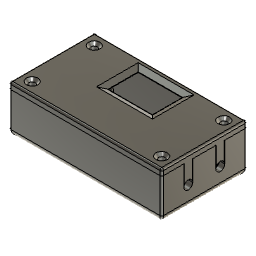
Controller_DC-DC_box (Autodesk Fusion 360 design; units mm, degrees)
Autodesk Fusion 360 part; units mm, degrees
sketch "Sketch1" plane through (0, 0, 0) normal (0, 0, 1) x (1, 0, 0)
  line L0 (-40, 21) -> (40, 21)
  line L1 (40, 21) -> (40, -21)
  line L2 (40, -21) -> (-40, -21)
  line L3 (-40, -21) -> (-40, 21)
  line L4 (1.75, 0) -> (22.5, 0)
  line L5 (0, 1.75) -> (0, 22.5)
  dimension "d1" = 80
  dimension "d2" = 42
  constraint horizontal L0
  constraint vertical L1
  constraint horizontal L2
  constraint vertical L3
  constraint symmetric L0 L2 L4
  constraint symmetric L1 L3 L5
  measures "d1" distance of L0.start L0.end
  measures "d2" distance of L0.start L2.end
extrude "Extrude1" add sketch "Sketch1" along normal blind 3 makes body 1
sketch "Sketch2" plane through (0, 0, 0) normal (0, 0, -1) x (1, 0, 0)
  line L0 (40, 21) -> (-40, 21)
  line L1 (-40, 21) -> (-40, -21)
  line L2 (-40, -21) -> (40, -21)
  line L3 (40, -21) -> (40, 21)
  line L4 (-43, -24) -> (43, -24)
  line L5 (43, -24) -> (43, 24)
  line L6 (43, 24) -> (-43, 24)
  line L7 (-43, 24) -> (-43, -24)
  dimension "d5" = 3
extrude "Extrude2" add sketch "Sketch2" against normal blind 23 bodies 1
sketch "Sketch3" plane through (0, 0, 3) normal (0, 0, 1) x (-1, 0, 0)
  line L0 (40, 21) -> (-40, 21)
  line L1 (-40, 21) -> (-40, -21)
  line L2 (-40, -21) -> (40, -21)
  line L3 (40, -21) -> (40, 21)
  line L4 (29, -16) -> (-29, -16) construction
  line L5 (-29, -16) -> (-29, 16) construction
  line L6 (-29, 16) -> (29, 16) construction
  line L7 (29, 16) -> (29, -16) construction
  line L8 (-1.75, 0) -> (-22.5, 0) construction
  line L9 (0, -1.75) -> (0, -22.5) construction
  circle A0 centre (29, -16) radius 3.5
  circle A1 centre (29, -16) radius 1.75
  circle A2 centre (-29, -16) radius 1.75
  circle A3 centre (-29, -16) radius 3.5
  circle A4 centre (-29, 16) radius 1.75
  circle A5 centre (-29, 16) radius 3.5
  circle A6 centre (29, 16) radius 1.75
  circle A7 centre (29, 16) radius 3.5
  dimension "d8" = 58
  dimension "d9" = 32
  dimension "d10" = 7
  dimension "d11" = 3.5
  constraint horizontal L4
  constraint vertical L5
  constraint horizontal L6
  constraint vertical L7
  constraint symmetric L4 L6 L8
  constraint symmetric L5 L7 L9
  constraint coincident L4.start L7.end
  constraint concentric A0 A1
  constraint coincident L4.end L5.start
  constraint concentric A2 A3
  constraint coincident L5.end L6.start
  constraint concentric A4 A5
  constraint coincident L6.end L7.start
  constraint concentric A6 A7
  constraint equal A1 A6
  constraint equal A1 A2
  constraint equal A1 A4
  constraint equal A0 A3
  constraint equal A0 A5
  constraint equal A0 A7
  measures "d8" distance of L4.start L4.end
  measures "d9" distance of L4.start L6.end
  measures "d10" diameter of A0
  measures "d11" diameter of A1
extrude "Extrude3" add sketch "Sketch3" along normal blind 6 contours A0 | A3 | A5 | A7 bodies 1
sketch "Sketch4" plane through (0, 0, 3) normal (0, 0, 1) x (-1, 0, 0)
  circle A0 centre (29, -16) radius 3.5
  circle A1 centre (-29, -16) radius 3.5
  line L0 (40, 21) -> (-40, 21)
  line L1 (-40, 21) -> (-40, -21)
  line L2 (-40, -21) -> (40, -21)
  line L3 (40, -21) -> (40, 21)
  circle A2 centre (-29, 16) radius 3.5
  circle A3 centre (29, 16) radius 3.5
  line L4 (40, 12.5) -> (33, 12.5)
  line L5 (33, 12.5) -> (33, -12.5)
  line L6 (33, -12.5) -> (40, -12.5)
  line L7 (40, -12.5) -> (40, 12.5)
  line L8 (-1.75, 0) -> (-22.5, 0)
  line L9 (0, -1.75) -> (0, -22.5)
  line L10 (-33, -12.5) -> (-40, -12.5)
  line L11 (-40, -12.5) -> (-40, 12.5)
  line L12 (-33, 12.5) -> (-33, -12.5)
  line L13 (-40, 12.5) -> (-33, 12.5)
  dimension "d14" = 7
  dimension "d15" = 25
  constraint horizontal L4
  constraint vertical L5
  constraint horizontal L6
  constraint vertical L7
  constraint coincident L3 L4.start
  constraint symmetric L4 L6 L8
  constraint symmetric L4.start L9 L11.end
  constraint symmetric L4.end L9 L12.start
  constraint symmetric L5.end L9 L10.start
  constraint symmetric L6.end L9 L10.end
  measures "d14" distance of L4.start L4.end
  measures "d15" distance of L4.start L6.end
extrude "Extrude4" add sketch "Sketch4" along normal blind 6 contours L3 L4 L5 L6 L7 | L1 L10 L11 L12 L13 bodies 1
sketch "Sketch5" plane through (-40, 0, 0) normal (1, 0, 0) x (0, 1, 0)
  line L0 (-12.5, 3) -> (-12.5, 9)
  line L1 (-12.5, 9) -> (12.5, 9)
  line L2 (12.5, 9) -> (12.5, 3)
  line L3 (12.5, 3) -> (21, 3)
  line L4 (21, 3) -> (21, 23)
  line L5 (21, 23) -> (-21, 23)
  line L6 (-21, 23) -> (-21, 3)
  line L7 (-21, 3) -> (-12.5, 3)
  circle A0 centre (-9, 11.5) radius 2.5
  circle A1 centre (9, 11.5) radius 2.5
  line L8 (0, 1.75) -> (0, 22.5)
  line L9 (-11.5, 11.5) -> (-11.5, 23)
  line L10 (-6.5, 11.5) -> (-6.5, 23)
  line L11 (-11.5, 23) -> (-6.5, 23)
  line L12 (6.5, 11.5) -> (6.5, 23)
  line L13 (6.5, 23) -> (11.5, 23)
  line L14 (11.5, 23) -> (11.5, 11.5)
  dimension "d18" = 5
  dimension "d19" = 9
  dimension "d20" = 18
  dimension "d24" = 5
  constraint equal A0 A1
  constraint horizontal A0.centre A1.centre
  constraint tangent L1 A0
  constraint coincident A0 L9.start
  constraint coincident L5 L9.end
  constraint tangent A0 L9
  constraint perpendicular L5 L9
  constraint coincident A0 L10.start
  constraint coincident L5 L10.end
  constraint tangent A0 L10
  constraint perpendicular L5 L10
  constraint coincident A1 L12.start
  constraint coincident L5 L12.end
  constraint tangent A1 L12
  constraint perpendicular L5 L12
  constraint perpendicular L12 L13
  constraint coincident A1 L14.end
  constraint tangent A1 L14
  measures "d18" diameter of A0
  measures "d19" distance of A0.centre L8
  measures "d20" distance of A0.centre A1.centre
  measures "d24" distance of L12.end L13.end
extrude "Extrude5" cut sketch "Sketch5" against normal through all contours A0 | L5 A0 L9 L10 L11 | A1 | L5 A1 L12 L13 L14 bodies 1
mirror "Mirror1" about plane through (0, 0, 0) normal (1, 0, 0) of "Extrude5"
extrude "Extrude7" add 1 faces at (40, 2.1667, 15.3333) along direction (-1, 0, 0) blind 3 on bodies 1 bodies 1
extrude "Extrude8" add 1 faces at (-40, 2.1667, 15.3333) along direction (1, 0, 0) blind 3 on bodies 1 bodies 1
sketch "Sketch7" plane through (0, 0, 23) normal (0, 0, 1) x (-1, 0, 0)
  line L0 (-40, -11.5) -> (-43, -11.5)
  line L1 (-43, -11.5) -> (-43, -24)
  line L2 (-43, -24) -> (43, -24)
  line L3 (43, -24) -> (43, -11.5)
  line L4 (43, -11.5) -> (40, -11.5)
  line L5 (40, -11.5) -> (40, -21)
  line L6 (40, -21) -> (-40, -21)
  line L7 (-40, -21) -> (-40, -11.5)
  line L8 (-40, 21) -> (-33, 21)
  line L9 (-33, 21) -> (-33, 14)
  line L10 (-33, 14) -> (-40, 14)
  line L11 (-40, 14) -> (-40, 21)
  circle A0 centre (-36.5, 17.5) radius 1.75
  line L12 (-40, 21) -> (40, 21)
  line L13 (-40, 11.5) -> (-40, 21)
  line L14 (-1.75, 0) -> (-22.5, 0)
  circle A1 centre (-36.5, -17.5) radius 1.75
  line L15 (-33, -21) -> (-33, -14)
  line L16 (-33, -14) -> (-40, -14)
  line L17 (-40, -14) -> (-40, -21)
  line L18 (-40, -21) -> (-33, -21)
  line L19 (0, -1.75) -> (0, -22.5)
  line L20 (33, -21) -> (33, -14)
  circle A2 centre (36.5, -17.5) radius 1.75
  line L21 (33, -14) -> (40, -14)
  line L22 (40, -14) -> (40, -21)
  line L23 (40, -21) -> (33, -21)
  line L24 (33, 21) -> (33, 14)
  line L25 (33, 14) -> (40, 14)
  line L26 (40, 14) -> (40, 21)
  line L27 (40, 21) -> (33, 21)
  circle A3 centre (36.5, 17.5) radius 1.75
  dimension "d31" = 7
  dimension "d32" = 7
  dimension "d33" = 3.5
  dimension "d34" = 3.5
  dimension "d72" = 3.5
  constraint horizontal L8
  constraint vertical L9
  constraint horizontal L10
  constraint vertical L11
  constraint coincident L8.start L12
  constraint coincident L8.start L13
  constraint symmetric L8.start L14 L6.end
  constraint symmetric L8.end L14 L15.start
  constraint symmetric L9.end L14 L15.end
  constraint symmetric L10.end L14 L16.end
  constraint symmetric A0 L14 A1
  constraint symmetric L8.start L19 L12.end
  constraint symmetric L8.end L19 L24.start
  constraint symmetric L9.end L19 L24.end
  constraint symmetric L10.end L19 L25.end
  constraint symmetric A0 L19 A3
  constraint symmetric A1 L19 A2
  constraint symmetric L15.start L19 L20.start
  constraint symmetric L15.end L19 L20.end
  constraint symmetric L16.end L19 L21.end
  constraint symmetric L6.end L19 L5.end
  measures "d31" distance of L8.start L10.end
  measures "d32" distance of L8.start L8.end
  measures "d33" distance of L11 A0.centre
  measures "d34" distance of L10 A0.centre
  measures "d72" diameter of A0
extrude "Extrude6" add sketch "Sketch7" against normal blind 6 contours L6 L7 L15 L16 L17 L18 | L5 L6 L20 L21 L22 L23 | L8 L9 L10 L11 L12 L13 | L12 L24 L25 L26 L27 bodies 1
fillet "Fillet3" radius 3.5 4 edges at (33, -14, 20) (-33, -14, 20) (-33, 14, 20) (33, 14, 20) on bodies 1
sketch "Sketch1 (2)" plane through (0, 0, 23) normal (0, 0, 1) x (-1, 0, 0) in component "Lid"
  circle A0 centre (-36.5, 17.5) radius 1.75
  circle A1 centre (36.5, 17.5) radius 1.75
  circle A2 centre (36.5, -17.5) radius 1.75
  circle A3 centre (-36.5, -17.5) radius 1.75
  line L0 (43, 24) -> (43, -24)
  line L1 (43, -24) -> (-43, -24)
  line L2 (-43, -24) -> (-43, 24)
  line L3 (-43, 24) -> (43, 24)
extrude "Extrude1'" add sketch "Sketch1 (2)" along normal blind 3.5 separate body makes body 2 in component "Lid"
sketch "Sketch2 (2)" plane through (-43, 0, 0) normal (-1, 0, 0) x (0, -1, 0) in component "Lid"
  line L0 (-11.5, 11.5) -> (-11.5, 24)
  line L1 (-6.5, 24) -> (-6.5, 11.5)
  arc A0 (-11.5, 11.5) -> (-6.5, 11.5) centre (-9, 11.5) ccw
  line L2 (-11.5, 11.5) -> (-11.5, 24)
  line L3 (-6.5, 11.5) -> (-6.5, 24)
  line L4 (-6.5, 24) -> (-11.5, 24)
  arc A1 (-6.5, 11.5) -> (-11.5, 11.5) centre (-9, 11.5) ccw
  line L5 (-11.3, 11.929) -> (-11.3, 24)
  line L6 (-6.7, 11.929) -> (-6.7, 24)
  line L7 (0, 1.75) -> (0, 22.5)
  arc A2 (-6.7397, 11.9253) -> (-11.2603, 11.9253) centre (-9, 11.5) ccw
  arc A3 (-11.3, 11.929) -> (-11.2603, 11.9253) centre (-11.28, 11.929) ccw
  arc A4 (-6.7397, 11.9253) -> (-6.7, 11.929) centre (-6.72, 11.929) ccw
  line L8 (24, 24) -> (-24, 24)
  line L9 (-24, 24) -> (-24, 28)
  line L10 (-24, 28) -> (24, 28)
  line L11 (24, 28) -> (24, 24)
  line L12 (-24, 23) -> (24, 23)
  line L13 (24, 23) -> (24, 26.5)
  line L14 (24, 26.5) -> (-24, 26.5)
  line L15 (-24, 26.5) -> (-24, 23)
  dimension "d69" = 0.02
  dimension "d75" = 0.2
  constraint concentric A0 A1
  constraint coincident L0.start A0.start
  constraint coincident L0.end L2.end
  constraint coincident L1.end A0.end
  constraint coincident L1.start L3.end
  constraint concentric A1 A2
  constraint tangent A2 A3
  constraint tangent L5 A3
  constraint tangent A2 A4
  constraint tangent L6 A4
  constraint equal A3 A4
  measures "d69" radius of A3
  measures "d75" distance of A1 A2
extrude "Extrude2'" add sketch "Sketch2 (2)" against normal blind 6 contours A1 L5 L6 L12 | L4 L5 L6 L8 L12 bodies 2 in component "Lid"
mirror "Mirror2" about plane through (0, 0, 0) normal (0, 1, 0) of "Extrude2'" in component "Lid"
mirror "Mirror1'" about plane through (0, 0, 0) normal (1, 0, 0) of "Extrude2'", "Mirror2" in component "Lid"
sketch "Sketch3 (2)" plane through (0, 0, 26.5) normal (0, 0, 1) x (-1, 0, 0) in component "Lid"
  line L0 (-43, 24) -> (-43, -24)
  line L1 (43, -24) -> (43, 24)
  line L2 (-12.5, -1.25) -> (12.5, -1.25)
  line L3 (12.5, -1.25) -> (12.5, -18.25)
  line L4 (12.5, -18.25) -> (-12.5, -18.25)
  line L5 (-12.5, -18.25) -> (-12.5, -1.25)
  line L6 (0, -1.75) -> (0, -22.5)
  circle A0 centre (-29, -16) radius 1.75
  circle A1 centre (29, -16) radius 1.75
  line L7 (29, -17.75) -> (-29, -17.75) construction
  circle A2 centre (36.5, -17.5) radius 1.75
  circle A3 centre (-36.5, 17.5) radius 1.75
  circle A4 centre (36.5, 17.5) radius 1.75
  circle A5 centre (-36.5, -17.5) radius 1.75
  line L8 (-43, -24) -> (43, -24)
  line L9 (43, 24) -> (-43, 24)
  dimension "d52" = 25
  dimension "d53" = 17
  dimension "d62" = 0.5
  constraint horizontal L2
  constraint vertical L3
  constraint horizontal L4
  constraint vertical L5
  constraint symmetric L3 L5 L6
  constraint coincident A1 L7.start
  constraint coincident A0 L7.end
  constraint tangent A0 L7
  measures "d52" distance of L2.start L2.end
  measures "d53" distance of L2.start L4.end
  measures "d62" distance of L4 L7
extrude "Extrude3'" cut sketch "Sketch3 (2)" against normal up to surface (3.5 mm away) contours L2 L3 L4 L5 bodies 2 in component "Lid"
sketch "Sketch4 (2)" plane through (0, 0, 23) normal (0, 0, -1) x (1, 0, 0) in component "Lid"
  line L0 (12.5, -1.25) -> (12.5, -18.25)
  line L1 (12.5, -18.25) -> (-12.5, -18.25)
  line L2 (-12.5, -18.25) -> (-12.5, -1.25)
  line L3 (-12.5, -1.25) -> (12.5, -1.25)
  line L4 (-43, 24) -> (-43, 11.3)
  line L5 (-43, -6.7) -> (-37, -6.7)
  line L6 (-37, -6.7) -> (-37, -11.3)
  line L7 (-37, -11.3) -> (-43, -11.3)
  line L8 (-43, -11.3) -> (-43, -24)
  line L9 (43, 11.3) -> (43, 24)
  line L10 (43, -11.3) -> (37, -11.3)
  line L11 (37, -11.3) -> (37, -6.7)
  line L12 (37, -6.7) -> (43, -6.7)
  line L13 (43, -6.7) -> (43, 6.7)
  line L14 (-14.5, 0.75) -> (14.5, 0.75)
  line L15 (14.5, 0.75) -> (14.5, -20.25)
  line L16 (14.5, -20.25) -> (-14.5, -20.25)
  line L17 (-14.5, -20.25) -> (-14.5, 0.75)
  line L18 (37, 11.3) -> (43, 11.3)
  line L19 (-43, 11.3) -> (-37, 11.3)
  line L20 (-37, 11.3) -> (-37, 6.7)
  line L21 (-37, 6.7) -> (-43, 6.7)
  line L22 (-43, 6.7) -> (-43, -6.7)
  line L23 (43, 6.7) -> (37, 6.7)
  line L24 (37, 6.7) -> (37, 11.3)
  line L25 (43, 24) -> (-43, 24)
  line L26 (-43, -24) -> (43, -24)
  line L27 (43, -24) -> (43, -11.3)
  circle A0 centre (-36.5, -17.5) radius 1.75
  circle A1 centre (36.5, 17.5) radius 1.75
  circle A2 centre (-36.5, 17.5) radius 1.75
  circle A3 centre (36.5, -17.5) radius 1.75
  dimension "d56" = -2
extrude "Extrude4'" cut sketch "Sketch4 (2)" against normal blind 2 contours L14 L15 L16 L17 bodies 2 in component "Lid"
chamfer "Chamfer1" distance 3.25 distance2 1.2 4 edges at (0, 1.25, 26.5) (12.5, 9.75, 26.5) (0, 18.25, 26.5) (-12.5, 9.75, 26.5) measured on face at (4.1667, -11.7562, 26.5) measured on face at (4.1667, -11.7562, 26.5) measured on face at (4.1667, -11.7562, 26.5) measured on face at (4.1667, -11.7562, 26.5) on bodies 2 in component "Lid"
chamfer "Chamfer3" distance 1.5 angle 45 4 edges at (-34.8684, 16.8672, 26.5) (-34.8684, -18.1328, 26.5) (38.1316, -18.1328, 26.5) (38.1316, 16.8672, 26.5) on bodies 2 in component "Lid"
chamfer "Chamfer2" distance 0.75 angle 45 8 edges at (38.1316, 16.8672, 23) (38.1316, -18.1328, 23) (-34.8684, -18.1328, 23) (-27.3684, -16.6328, 9) (-27.3684, 15.3672, 9) (-34.8684, 16.8672, 23) (30.6316, 15.3672, 9) (30.6316, -16.6328, 9) on bodies 1
fillet "Fillet4" radius 1 4 edges at (43, -24, 11.5) (-43, -24, 11.5) (43, 24, 11.5) (-43, 24, 11.5) on bodies 1
fillet "Fillet2" radius 1 8 edges at (0, -24, 26.5) (43, -24, 24.75) (-43, -24, 24.75) (-43, 0, 26.5) (0, 24, 26.5) (43, 0, 26.5) (43, 24, 24.75) (-43, 24, 24.75) on bodies 2 in component "Lid"
fillet "Fillet5" radius 3.5 8 edges at (42.7071, 23.7071, 0) (43, 0, 0) (42.7071, -23.7071, 0) (0, -24, 0) (-42.7071, -23.7071, 0) (-43, 0, 0) (-42.7071, 23.7071, 0) (0, 24, 0) on bodies 1
sketch "Sketch5 (2)" plane through (0, 0, 23) normal (0, 0, -1) x (1, 0, 0) in component "Lid"
  arc A0 (42, -24) -> (43, -23) centre (42, -23) ccw
  line L0 (43, -23) -> (43, -11.3)
  line L1 (43, -11.3) -> (37, -11.3)
  line L2 (37, -11.3) -> (37, -6.7)
  line L3 (37, -6.7) -> (43, -6.7)
  line L4 (43, -6.7) -> (43, 6.7)
  line L5 (43, 6.7) -> (37, 6.7)
  line L6 (37, 6.7) -> (37, 11.3)
  line L7 (37, 11.3) -> (43, 11.3)
  line L8 (43, 11.3) -> (43, 23)
  arc A1 (43, 23) -> (42, 24) centre (42, 23) ccw
  line L9 (42, 24) -> (-42, 24)
  arc A2 (-42, 24) -> (-43, 23) centre (-42, 23) ccw
  line L10 (-43, 23) -> (-43, 11.3)
  line L11 (-43, 11.3) -> (-37, 11.3)
  line L12 (-37, 11.3) -> (-37, 6.7)
  line L13 (-37, 6.7) -> (-43, 6.7)
  line L14 (-43, 6.7) -> (-43, -6.7)
  line L15 (-43, -6.7) -> (-37, -6.7)
  line L16 (-37, -6.7) -> (-37, -11.3)
  line L17 (-37, -11.3) -> (-43, -11.3)
  line L18 (-43, -11.3) -> (-43, -23)
  arc A3 (-43, -23) -> (-42, -24) centre (-42, -23) ccw
  line L19 (-42, -24) -> (42, -24)
  line L20 (14.5, 0.75) -> (14.5, -20.25)
  line L21 (14.5, -20.25) -> (-14.5, -20.25)
  line L22 (-14.5, -20.25) -> (-14.5, 0.75)
  line L23 (-14.5, 0.75) -> (14.5, 0.75)
  circle A4 centre (36.5, 17.5) radius 1.75
  circle A5 centre (36.5, -17.5) radius 1.75
  circle A6 centre (-36.5, -17.5) radius 1.75
  circle A7 centre (-36.5, 17.5) radius 1.75
  circle A8 centre (-7, 15) radius 2
  dimension "d84" = 4
  dimension "d85" = 36
  dimension "d86" = 9
  measures "d84" diameter of A8
  measures "d85" distance of L10 A8.centre
  measures "d86" distance of L9 A8.centre
extrude "Extrude5'" cut sketch "Sketch5 (2)" against normal blind 1.5 contours A8 bodies 2 in component "Lid"
fillet "Fillet3'" radius 1 1 edges at (-8.8647, -15.7232, 24.5) on bodies 2 in component "Lid"
component "Lid" placed x (1, 0, 0) y (0, 1, 0) z (0, 0, 1) at (0, 0, 0)
equation "d19 = d20 / 2"
equation "d26 = d27"
equation "d27 = 7 mm"
equation "d29 = d27 / 2"
equation "d30 = d26 / 2"
equation "d31 = d27"
equation "d32 = d26"
equation "d33 = d30"
equation "d34 = d29"
